Autodesk Inventor part; units mm, degrees
(part 3 of 3)
  arc A136 (-306.3004, -73.6879) -> (-305.5933, -73.9808) centre (-305.5933, -72.9808) ccw
  arc A137 (-305.5933, -68.9808) -> (-306.3004, -69.2736) centre (-305.5933, -69.9808) ccw
  line L344 (-306.3004, -73.6879) -> (-308.2075, -71.7808)
  line L345 (-306.3004, -69.2736) -> (-308.2075, -71.1808)
  line L346 (-308.2075, -71.4808) -> (-308.2075, -71.7808)
  line L347 (-308.2075, -71.4808) -> (-308.2075, -71.1808)
  line L348 (-305.5933, -68.9808) -> (-288.8217, -68.9808)
  line L349 (-288.8217, -73.9808) -> (-305.5933, -73.9808)
  arc A138 (-288.1146, -69.2736) -> (-288.8217, -68.9808) centre (-288.8217, -69.9808) ccw
  line L350 (-288.1146, -69.2736) -> (-286.2075, -71.1808)
  line L351 (-286.2075, -71.4808) -> (-286.2075, -71.1808)
  line L352 (-286.2075, -71.4808) -> (-286.2075, -71.7808)
  arc A139 (-288.8217, -73.9808) -> (-288.1146, -73.6879) centre (-288.8217, -72.9808) ccw
  line L353 (-288.1146, -73.6879) -> (-286.2075, -71.7808)
  arc A140 (-100.8004, -24.0879) -> (-100.0933, -24.3808) centre (-100.0933, -23.3808) ccw
  arc A141 (-100.0933, -19.3808) -> (-100.8004, -19.6736) centre (-100.0933, -20.3808) ccw
  line L354 (-100.8004, -24.0879) -> (-102.7075, -22.1808)
  line L355 (-100.8004, -19.6736) -> (-102.7075, -21.5808)
  line L356 (-102.7075, -21.8808) -> (-102.7075, -22.1808)
  line L357 (-102.7075, -21.8808) -> (-102.7075, -21.5808)
  line L358 (-100.0933, -19.3808) -> (-83.3217, -19.3808)
  line L359 (-83.3217, -24.3808) -> (-100.0933, -24.3808)
  arc A142 (-82.6146, -19.6736) -> (-83.3217, -19.3808) centre (-83.3217, -20.3808) ccw
  line L360 (-82.6146, -19.6736) -> (-80.7075, -21.5808)
  line L361 (-80.7075, -21.8808) -> (-80.7075, -21.5808)
  line L362 (-80.7075, -21.8808) -> (-80.7075, -22.1808)
  arc A143 (-83.3217, -24.3808) -> (-82.6146, -24.0879) centre (-83.3217, -23.3808) ccw
  line L363 (-82.6146, -24.0879) -> (-80.7075, -22.1808)
  arc A144 (-100.8004, -48.8879) -> (-100.0933, -49.1808) centre (-100.0933, -48.1808) ccw
  arc A145 (-100.0933, -44.1808) -> (-100.8004, -44.4736) centre (-100.0933, -45.1808) ccw
  line L364 (-100.8004, -48.8879) -> (-102.7075, -46.9808)
  line L365 (-100.8004, -44.4736) -> (-102.7075, -46.3808)
  line L366 (-102.7075, -46.6808) -> (-102.7075, -46.9808)
  line L367 (-102.7075, -46.6808) -> (-102.7075, -46.3808)
  line L368 (-100.0933, -44.1808) -> (-83.3217, -44.1808)
  line L369 (-83.3217, -49.1808) -> (-100.0933, -49.1808)
  arc A146 (-82.6146, -44.4736) -> (-83.3217, -44.1808) centre (-83.3217, -45.1808) ccw
  line L370 (-82.6146, -44.4736) -> (-80.7075, -46.3808)
  line L371 (-80.7075, -46.6808) -> (-80.7075, -46.3808)
  line L372 (-80.7075, -46.6808) -> (-80.7075, -46.9808)
  arc A147 (-83.3217, -49.1808) -> (-82.6146, -48.8879) centre (-83.3217, -48.1808) ccw
  line L373 (-82.6146, -48.8879) -> (-80.7075, -46.9808)
  arc A148 (-101.9004, -43.3736) -> (-101.6075, -42.6665) centre (-102.6075, -42.6665) ccw
  arc A149 (-106.6075, -42.6665) -> (-106.3146, -43.3736) centre (-105.6075, -42.6665) ccw
  line L374 (-101.9004, -43.3736) -> (-103.8075, -45.2808)
  line L375 (-106.3146, -43.3736) -> (-104.4075, -45.2808)
  line L376 (-104.1075, -45.2808) -> (-103.8075, -45.2808)
  line L377 (-104.1075, -45.2808) -> (-104.4075, -45.2808)
  line L378 (-106.6075, -42.6665) -> (-106.6075, -25.895)
  line L379 (-101.6075, -25.895) -> (-101.6075, -42.6665)
  arc A150 (-106.3146, -25.1879) -> (-106.6075, -25.895) centre (-105.6075, -25.895) ccw
  line L380 (-106.3146, -25.1879) -> (-104.4075, -23.2808)
  line L381 (-104.1075, -23.2808) -> (-104.4075, -23.2808)
  line L382 (-104.1075, -23.2808) -> (-103.8075, -23.2808)
  arc A151 (-101.6075, -25.895) -> (-101.9004, -25.1879) centre (-102.6075, -25.895) ccw
  line L383 (-101.9004, -25.1879) -> (-103.8075, -23.2808)
  arc A152 (-101.9004, -68.1736) -> (-101.6075, -67.4665) centre (-102.6075, -67.4665) ccw
  arc A153 (-106.6075, -67.4665) -> (-106.3146, -68.1736) centre (-105.6075, -67.4665) ccw
  line L384 (-101.9004, -68.1736) -> (-103.8075, -70.0808)
  line L385 (-106.3146, -68.1736) -> (-104.4075, -70.0808)
  line L386 (-104.1075, -70.0808) -> (-103.8075, -70.0808)
  line L387 (-104.1075, -70.0808) -> (-104.4075, -70.0808)
  line L388 (-106.6075, -67.4665) -> (-106.6075, -50.695)
  line L389 (-101.6075, -50.695) -> (-101.6075, -67.4665)
  arc A154 (-106.3146, -49.9879) -> (-106.6075, -50.695) centre (-105.6075, -50.695) ccw
  line L390 (-106.3146, -49.9879) -> (-104.4075, -48.0808)
  line L391 (-104.1075, -48.0808) -> (-104.4075, -48.0808)
  line L392 (-104.1075, -48.0808) -> (-103.8075, -48.0808)
  arc A155 (-101.6075, -50.695) -> (-101.9004, -49.9879) centre (-102.6075, -50.695) ccw
  line L393 (-101.9004, -49.9879) -> (-103.8075, -48.0808)
  arc A156 (-77.1004, -43.3736) -> (-76.8075, -42.6665) centre (-77.8075, -42.6665) ccw
  arc A157 (-81.8075, -42.6665) -> (-81.5146, -43.3736) centre (-80.8075, -42.6665) ccw
  line L394 (-77.1004, -43.3736) -> (-79.0075, -45.2808)
  line L395 (-81.5146, -43.3736) -> (-79.6075, -45.2808)
  line L396 (-79.3075, -45.2808) -> (-79.0075, -45.2808)
  line L397 (-79.3075, -45.2808) -> (-79.6075, -45.2808)
  line L398 (-81.8075, -42.6665) -> (-81.8075, -25.895)
  line L399 (-76.8075, -25.895) -> (-76.8075, -42.6665)
  arc A158 (-81.5146, -25.1879) -> (-81.8075, -25.895) centre (-80.8075, -25.895) ccw
  line L400 (-81.5146, -25.1879) -> (-79.6075, -23.2808)
  line L401 (-79.3075, -23.2808) -> (-79.6075, -23.2808)
  line L402 (-79.3075, -23.2808) -> (-79.0075, -23.2808)
  arc A159 (-76.8075, -25.895) -> (-77.1004, -25.1879) centre (-77.8075, -25.895) ccw
  line L403 (-77.1004, -25.1879) -> (-79.0075, -23.2808)
  arc A160 (-77.1004, -68.1736) -> (-76.8075, -67.4665) centre (-77.8075, -67.4665) ccw
  arc A161 (-81.8075, -67.4665) -> (-81.5146, -68.1736) centre (-80.8075, -67.4665) ccw
  line L404 (-77.1004, -68.1736) -> (-79.0075, -70.0808)
  line L405 (-81.5146, -68.1736) -> (-79.6075, -70.0808)
  line L406 (-79.3075, -70.0808) -> (-79.0075, -70.0808)
  line L407 (-79.3075, -70.0808) -> (-79.6075, -70.0808)
  line L408 (-81.8075, -67.4665) -> (-81.8075, -50.695)
  line L409 (-76.8075, -50.695) -> (-76.8075, -67.4665)
  arc A162 (-81.5146, -49.9879) -> (-81.8075, -50.695) centre (-80.8075, -50.695) ccw
  line L410 (-81.5146, -49.9879) -> (-79.6075, -48.0808)
  line L411 (-79.3075, -48.0808) -> (-79.6075, -48.0808)
  line L412 (-79.3075, -48.0808) -> (-79.0075, -48.0808)
  arc A163 (-76.8075, -50.695) -> (-77.1004, -49.9879) centre (-77.8075, -50.695) ccw
  line L413 (-77.1004, -49.9879) -> (-79.0075, -48.0808)
  arc A164 (-100.8004, -73.6879) -> (-100.0933, -73.9808) centre (-100.0933, -72.9808) ccw
  arc A165 (-100.0933, -68.9808) -> (-100.8004, -69.2736) centre (-100.0933, -69.9808) ccw
  line L414 (-100.8004, -73.6879) -> (-102.7075, -71.7808)
  line L415 (-100.8004, -69.2736) -> (-102.7075, -71.1808)
  line L416 (-102.7075, -71.4808) -> (-102.7075, -71.7808)
  line L417 (-102.7075, -71.4808) -> (-102.7075, -71.1808)
  line L418 (-100.0933, -68.9808) -> (-83.3217, -68.9808)
  line L419 (-83.3217, -73.9808) -> (-100.0933, -73.9808)
  arc A166 (-82.6146, -69.2736) -> (-83.3217, -68.9808) centre (-83.3217, -69.9808) ccw
  line L420 (-82.6146, -69.2736) -> (-80.7075, -71.1808)
  line L421 (-80.7075, -71.4808) -> (-80.7075, -71.1808)
  line L422 (-80.7075, -71.4808) -> (-80.7075, -71.7808)
  arc A167 (-83.3217, -73.9808) -> (-82.6146, -73.6879) centre (-83.3217, -72.9808) ccw
  line L423 (-82.6146, -73.6879) -> (-80.7075, -71.7808)
  line L424 (-237.0075, -35.3808) -> (-236.0075, -35.3808)
  line L425 (-236.0075, -35.3808) -> (-234.0075, -37.3808)
  line L426 (-234.0075, -37.3808) -> (-234.0075, -38.3808)
  line L427 (-234.0075, -38.3808) -> (-236.0075, -40.3808)
  line L428 (-236.0075, -40.3808) -> (-237.0075, -40.3808)
  line L429 (-237.0075, -40.3808) -> (-239.0075, -38.3808)
  line L430 (-239.0075, -38.3808) -> (-239.0075, -37.3808)
  line L431 (-239.0075, -37.3808) -> (-237.0075, -35.3808)
  line L432 (-237.0075, -55.3808) -> (-236.0075, -55.3808)
  line L433 (-236.0075, -55.3808) -> (-234.0075, -57.3808)
  line L434 (-234.0075, -57.3808) -> (-234.0075, -58.3808)
  line L435 (-234.0075, -58.3808) -> (-236.0075, -60.3808)
  line L436 (-236.0075, -60.3808) -> (-237.0075, -60.3808)
  line L437 (-237.0075, -60.3808) -> (-239.0075, -58.3808)
  line L438 (-239.0075, -58.3808) -> (-239.0075, -57.3808)
  line L439 (-239.0075, -57.3808) -> (-237.0075, -55.3808)
  line L440 (-152.9075, -35.3808) -> (-151.9075, -35.3808)
  line L441 (-151.9075, -35.3808) -> (-149.9075, -37.3808)
  line L442 (-149.9075, -37.3808) -> (-149.9075, -38.3808)
  line L443 (-149.9075, -38.3808) -> (-151.9075, -40.3808)
  line L444 (-151.9075, -40.3808) -> (-152.9075, -40.3808)
  line L445 (-152.9075, -40.3808) -> (-154.9075, -38.3808)
  line L446 (-154.9075, -38.3808) -> (-154.9075, -37.3808)
  line L447 (-154.9075, -37.3808) -> (-152.9075, -35.3808)
  line L448 (-152.9075, -55.3808) -> (-151.9075, -55.3808)
  line L449 (-151.9075, -55.3808) -> (-149.9075, -57.3808)
  line L450 (-149.9075, -57.3808) -> (-149.9075, -58.3808)
  line L451 (-149.9075, -58.3808) -> (-151.9075, -60.3808)
  line L452 (-151.9075, -60.3808) -> (-152.9075, -60.3808)
  line L453 (-152.9075, -60.3808) -> (-154.9075, -58.3808)
  line L454 (-154.9075, -58.3808) -> (-154.9075, -57.3808)
  line L455 (-154.9075, -57.3808) -> (-152.9075, -55.3808)
  arc A168 (-334.7004, -49.0879) -> (-333.9933, -49.3808) centre (-333.9933, -48.3808) ccw
  arc A169 (-333.9933, -44.3808) -> (-334.7004, -44.6736) centre (-333.9933, -45.3808) ccw
  line L456 (-334.7004, -49.0879) -> (-336.6075, -47.1808)
  line L457 (-336.6075, -46.8808) -> (-336.6075, -46.5808)
  line L458 (-336.6075, -46.8808) -> (-336.6075, -47.1808)
  line L459 (-334.7004, -44.6736) -> (-336.6075, -46.5808)
  line L460 (-333.9933, -44.3808) -> (-323.2217, -44.3808)
  line L461 (-323.2217, -49.3808) -> (-333.9933, -49.3808)
  arc A170 (-322.5146, -44.6736) -> (-323.2217, -44.3808) centre (-323.2217, -45.3808) ccw
  arc A171 (-323.2217, -49.3808) -> (-322.5146, -49.0879) centre (-323.2217, -48.3808) ccw
  line L462 (-322.5146, -49.0879) -> (-320.6075, -47.1808)
  line L463 (-320.6075, -46.8808) -> (-320.6075, -47.1808)
  line L464 (-320.6075, -46.8808) -> (-320.6075, -46.5808)
  line L465 (-322.5146, -44.6736) -> (-320.6075, -46.5808)
  arc A172 (-335.4004, -43.9736) -> (-335.1075, -43.2665) centre (-336.1075, -43.2665) ccw
  arc A173 (-340.1075, -43.2665) -> (-339.8146, -43.9736) centre (-339.1075, -43.2665) ccw
  line L466 (-335.4004, -43.9736) -> (-337.3075, -45.8808)
  line L467 (-337.6075, -45.8808) -> (-337.9075, -45.8808)
  line L468 (-337.6075, -45.8808) -> (-337.3075, -45.8808)
  line L469 (-339.8146, -43.9736) -> (-337.9075, -45.8808)
  line L470 (-340.1075, -43.2665) -> (-340.1075, -32.495)
  line L471 (-335.1075, -32.495) -> (-335.1075, -43.2665)
  arc A174 (-339.8146, -31.7879) -> (-340.1075, -32.495) centre (-339.1075, -32.495) ccw
  arc A175 (-335.1075, -32.495) -> (-335.4004, -31.7879) centre (-336.1075, -32.495) ccw
  line L472 (-335.4004, -31.7879) -> (-337.3075, -29.8808)
  line L473 (-337.6075, -29.8808) -> (-337.3075, -29.8808)
  line L474 (-337.6075, -29.8808) -> (-337.9075, -29.8808)
  line L475 (-339.8146, -31.7879) -> (-337.9075, -29.8808)
  arc A176 (-352.7004, -49.0879) -> (-351.9933, -49.3808) centre (-351.9933, -48.3808) ccw
  arc A177 (-351.9933, -44.3808) -> (-352.7004, -44.6736) centre (-351.9933, -45.3808) ccw
  line L476 (-352.7004, -49.0879) -> (-354.6075, -47.1808)
  line L477 (-354.6075, -46.8808) -> (-354.6075, -46.5808)
  line L478 (-354.6075, -46.8808) -> (-354.6075, -47.1808)
  line L479 (-352.7004, -44.6736) -> (-354.6075, -46.5808)
  line L480 (-351.9933, -44.3808) -> (-341.2217, -44.3808)
  line L481 (-341.2217, -49.3808) -> (-351.9933, -49.3808)
  arc A178 (-340.5146, -44.6736) -> (-341.2217, -44.3808) centre (-341.2217, -45.3808) ccw
  arc A179 (-341.2217, -49.3808) -> (-340.5146, -49.0879) centre (-341.2217, -48.3808) ccw
  line L482 (-340.5146, -49.0879) -> (-338.6075, -47.1808)
  line L483 (-338.6075, -46.8808) -> (-338.6075, -47.1808)
  line L484 (-338.6075, -46.8808) -> (-338.6075, -46.5808)
  line L485 (-340.5146, -44.6736) -> (-338.6075, -46.5808)
  arc A180 (-335.4004, -61.9736) -> (-335.1075, -61.2665) centre (-336.1075, -61.2665) ccw
  arc A181 (-340.1075, -61.2665) -> (-339.8146, -61.9736) centre (-339.1075, -61.2665) ccw
  line L486 (-335.4004, -61.9736) -> (-337.3075, -63.8808)
  line L487 (-337.6075, -63.8808) -> (-337.9075, -63.8808)
  line L488 (-337.6075, -63.8808) -> (-337.3075, -63.8808)
  line L489 (-339.8146, -61.9736) -> (-337.9075, -63.8808)
  line L490 (-340.1075, -61.2665) -> (-340.1075, -50.495)
  line L491 (-335.1075, -50.495) -> (-335.1075, -61.2665)
  arc A182 (-339.8146, -49.7879) -> (-340.1075, -50.495) centre (-339.1075, -50.495) ccw
  arc A183 (-335.1075, -50.495) -> (-335.4004, -49.7879) centre (-336.1075, -50.495) ccw
  line L492 (-335.4004, -49.7879) -> (-337.3075, -47.8808)
  line L493 (-337.6075, -47.8808) -> (-337.3075, -47.8808)
  line L494 (-337.6075, -47.8808) -> (-337.9075, -47.8808)
  line L495 (-339.8146, -49.7879) -> (-337.9075, -47.8808)
  arc A184 (-363.2004, -33.0879) -> (-362.4933, -33.3808) centre (-362.4933, -32.3808) ccw
  arc A185 (-362.4933, -28.3808) -> (-363.2004, -28.6736) centre (-362.4933, -29.3808) ccw
  line L496 (-363.2004, -33.0879) -> (-365.1075, -31.1808)
  line L497 (-365.1075, -30.8808) -> (-365.1075, -30.5808)
  line L498 (-365.1075, -30.8808) -> (-365.1075, -31.1808)
  line L499 (-363.2004, -28.6736) -> (-365.1075, -30.5808)
  line L500 (-362.4933, -28.3808) -> (-351.7217, -28.3808)
  line L501 (-351.7217, -33.3808) -> (-362.4933, -33.3808)
  arc A186 (-351.0146, -28.6736) -> (-351.7217, -28.3808) centre (-351.7217, -29.3808) ccw
  arc A187 (-351.7217, -33.3808) -> (-351.0146, -33.0879) centre (-351.7217, -32.3808) ccw
  line L502 (-351.0146, -33.0879) -> (-349.1075, -31.1808)
  line L503 (-349.1075, -30.8808) -> (-349.1075, -31.1808)
  line L504 (-349.1075, -30.8808) -> (-349.1075, -30.5808)
  line L505 (-351.0146, -28.6736) -> (-349.1075, -30.5808)
  arc A188 (-380.2004, -33.0879) -> (-379.4933, -33.3808) centre (-379.4933, -32.3808) ccw
  arc A189 (-379.4933, -28.3808) -> (-380.2004, -28.6736) centre (-379.4933, -29.3808) ccw
  line L506 (-380.2004, -33.0879) -> (-382.1075, -31.1808)
  line L507 (-382.1075, -30.8808) -> (-382.1075, -30.5808)
  line L508 (-382.1075, -30.8808) -> (-382.1075, -31.1808)
  line L509 (-380.2004, -28.6736) -> (-382.1075, -30.5808)
  line L510 (-379.4933, -28.3808) -> (-368.7217, -28.3808)
  line L511 (-368.7217, -33.3808) -> (-379.4933, -33.3808)
  arc A190 (-368.0146, -28.6736) -> (-368.7217, -28.3808) centre (-368.7217, -29.3808) ccw
  arc A191 (-368.7217, -33.3808) -> (-368.0146, -33.0879) centre (-368.7217, -32.3808) ccw
  line L512 (-368.0146, -33.0879) -> (-366.1075, -31.1808)
  line L513 (-366.1075, -30.8808) -> (-366.1075, -31.1808)
  line L514 (-366.1075, -30.8808) -> (-366.1075, -30.5808)
  line L515 (-368.0146, -28.6736) -> (-366.1075, -30.5808)
  arc A192 (-363.4004, -46.4879) -> (-363.1075, -45.7808) centre (-364.1075, -45.7808) ccw
  arc A193 (-368.1075, -45.7808) -> (-367.8146, -46.4879) centre (-367.1075, -45.7808) ccw
  line L516 (-363.4004, -46.4879) -> (-365.3075, -48.395)
  line L517 (-365.6075, -48.395) -> (-365.9075, -48.395)
  line L518 (-365.6075, -48.395) -> (-365.3075, -48.395)
  line L519 (-367.8146, -46.4879) -> (-365.9075, -48.395)
  line L520 (-368.1075, -45.7808) -> (-368.1075, -35.0092)
  line L521 (-363.1075, -35.0092) -> (-363.1075, -45.7808)
  arc A194 (-367.8146, -34.3021) -> (-368.1075, -35.0092) centre (-367.1075, -35.0092) ccw
  arc A195 (-363.1075, -35.0092) -> (-363.4004, -34.3021) centre (-364.1075, -35.0092) ccw
  line L522 (-363.4004, -34.3021) -> (-365.3075, -32.395)
  line L523 (-365.6075, -32.395) -> (-365.3075, -32.395)
  line L524 (-365.6075, -32.395) -> (-365.9075, -32.395)
  line L525 (-367.8146, -34.3021) -> (-365.9075, -32.395)
  arc A196 (-363.4004, -62.9879) -> (-363.1075, -62.2808) centre (-364.1075, -62.2808) ccw
  arc A197 (-368.1075, -62.2808) -> (-367.8146, -62.9879) centre (-367.1075, -62.2808) ccw
  line L526 (-363.4004, -62.9879) -> (-365.3075, -64.895)
  line L527 (-365.6075, -64.895) -> (-365.9075, -64.895)
  line L528 (-365.6075, -64.895) -> (-365.3075, -64.895)
  line L529 (-367.8146, -62.9879) -> (-365.9075, -64.895)
  line L530 (-368.1075, -62.2808) -> (-368.1075, -51.5092)
  line L531 (-363.1075, -51.5092) -> (-363.1075, -62.2808)
  arc A198 (-367.8146, -50.8021) -> (-368.1075, -51.5092) centre (-367.1075, -51.5092) ccw
  arc A199 (-363.1075, -51.5092) -> (-363.4004, -50.8021) centre (-364.1075, -51.5092) ccw
  line L532 (-363.4004, -50.8021) -> (-365.3075, -48.895)
  line L533 (-365.6075, -48.895) -> (-365.3075, -48.895)
  line L534 (-365.6075, -48.895) -> (-365.9075, -48.895)
  line L535 (-367.8146, -50.8021) -> (-365.9075, -48.895)
  point P0 (0, 0)
  dimension "d525" = 8
  dimension "d526" = 7.4
  dimension "d527" = 22
  dimension "d528" = 16.7
  dimension "d529" = 8
extrude "Extrusion3" cut sketch "Sketch5" against normal blind 3
body "Solid1"
